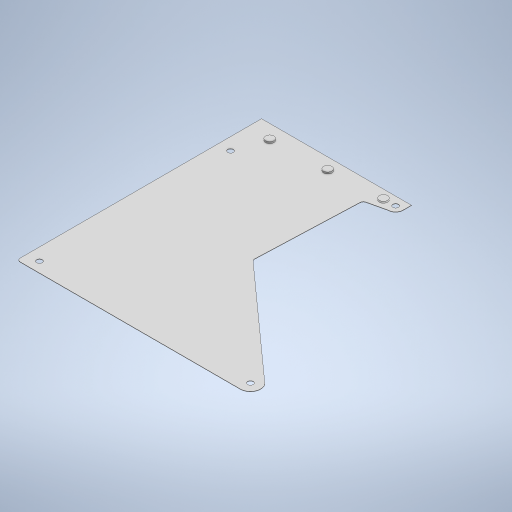
# Autodesk Inventor part: base_main_pcb_p1_itr2
Saved by Autodesk Inventor 2024 (Build 280153000, 153)
## iProperties
Created: 2026-03-21
Part Number: base_main_pcb_p1_itr2
Material: Generic
Document SubType Name: Modeling
Designer: schar
Density: 1 g/cm^3
Appearance: Default
Author: schar
Autodesk Inventor part; units mm, degrees
ref_plane "YZ Plane" through (0, 0, 0) normal (1, 0, 0) x (0, 1, 0)
ref_plane "XZ Plane" through (0, 0, 0) normal (0, 1, 0) x (-1, 0, 0)
ref_plane "XY Plane" through (0, 0, 0) normal (0, 0, 1) x (1, 0, 0)
ref_plane "Work Plane1" through (-203, 0.4, 290) normal (0, 1, 0) x (1, 0, 0)
sketch "Sketch1" plane through (-203, 0.4, 290) normal (0, 1, 0) x (1, 0, 0)
  arc A0 (133.6, 0) -> (138.4129, 10.1472) centre (133.6, 6.215) ccw projected
  circle A1 centre (133.6, 6.215) radius 1.675 projected
  circle A2 centre (133.6, 6.215) radius 1.675 projected
  circle A3 centre (133.6, 6.215) radius 1.675 projected
  circle A4 centre (133.6, 6.215) radius 1.675 projected
  arc A5 (133.6, 0) -> (138.4129, 10.1472) centre (133.6, 6.215) ccw projected
  arc A6 (133.6, 0) -> (138.4129, 10.1472) centre (133.6, 6.215) ccw projected
  arc A7 (133.6, 0) -> (138.4129, 10.1472) centre (133.6, 6.215) ccw projected
  circle A8 centre (84.5, 143.475) radius 1.675 projected
  arc A9 (84.5, 138.975) -> (89, 143.475) centre (84.5, 143.475) ccw projected
  arc A10 (73.455, 136.4093) -> (71.909, 134.5363) centre (73.9075, 134.4612) ccw projected
  arc A11 (73.455, 136.4093) -> (71.909, 134.5363) centre (73.9075, 134.4612) ccw projected
  circle A12 centre (5.5, 122.225) radius 1.675 projected
  circle A13 centre (5.5, 122.225) radius 1.675 projected
  circle A14 centre (5.5, 122.225) radius 1.675 projected
  circle A15 centre (5.5, 122.225) radius 1.675 projected
  line L0 (69.5853, 72.7034) -> (71.909, 134.5363) projected
  line L1 (69.5853, 72.7034) -> (71.909, 134.5363) projected
  line L2 (69.5853, 72.7034) -> (71.909, 134.5363) projected
  line L3 (69.5853, 72.7034) -> (71.909, 134.5363) projected
  circle A16 centre (5.5, 6.215) radius 1.675 projected
  line L4 (0, 0) -> (133.6, 0) projected
  line L5 (0, 0) -> (133.6, 0) projected
  line L6 (0, 0) -> (133.6, 0) projected
  line L7 (0, 0) -> (133.6, 0) projected
  line L8 (138.4129, 10.1472) -> (70.2502, 71.1379) projected
  line L9 (138.4129, 10.1472) -> (70.2502, 71.1379) projected
  line L10 (138.4129, 10.1472) -> (70.2502, 71.1379) projected
  line L11 (138.4129, 10.1472) -> (70.2502, 71.1379) projected
  arc A17 (73.455, 136.4093) -> (71.909, 134.5363) centre (73.9075, 134.4612) ccw projected
  arc A18 (73.455, 136.4093) -> (71.909, 134.5363) centre (73.9075, 134.4612) ccw projected
  circle A19 centre (5.5, 6.215) radius 1.675 projected
  arc A20 (-2, 2) -> (0, 0) centre (0, 2) ccw projected
  arc A21 (-2, 2) -> (0, 0) centre (0, 2) ccw projected
  arc A22 (-2, 2) -> (0, 0) centre (0, 2) ccw projected
  arc A23 (-2, 2) -> (0, 0) centre (0, 2) ccw projected
  circle A24 centre (5.5, 6.215) radius 1.675 projected
  circle A25 centre (5.5, 6.215) radius 1.675 projected
  arc A26 (69.5853, 72.7034) -> (70.2502, 71.1379) centre (71.5839, 72.6283) ccw projected
  arc A27 (69.5853, 72.7034) -> (70.2502, 71.1379) centre (71.5839, 72.6283) ccw projected
  arc A28 (69.5853, 72.7034) -> (70.2502, 71.1379) centre (71.5839, 72.6283) ccw projected
  arc A29 (69.5853, 72.7034) -> (70.2502, 71.1379) centre (71.5839, 72.6283) ccw projected
  arc A30 (84.5, 138.975) -> (89, 143.475) centre (84.5, 143.475) ccw projected
  circle A31 centre (84.5, 143.475) radius 1.675 projected
  circle A32 centre (84.5, 143.475) radius 1.675 projected
  circle A33 centre (84.5, 143.475) radius 1.675 projected
  arc A34 (84.5, 138.975) -> (89, 143.475) centre (84.5, 143.475) ccw projected
  arc A35 (84.5, 138.975) -> (89, 143.475) centre (84.5, 143.475) ccw projected
  line L12 (73.455, 136.4093) -> (84.5, 138.975) projected
  line L13 (73.455, 136.4093) -> (84.5, 138.975) projected
  line L14 (73.455, 136.4093) -> (84.5, 138.975) projected
  line L15 (73.455, 136.4093) -> (84.5, 138.975) projected
  line L16 (-2, 2) -> (-2, 148.562)
  line L17 (-2, 272.9952) -> (-2, 2) projected
  line L18 (-2, 148.562) -> (89, 148.562)
  line L19 (89, 143.475) -> (89, 199.525) projected
  line L20 (89, 148.562) -> (89, 143.475)
  point P0 (203, 290)
  point P1 (-2, 2)
  constraints: 6 end point, 3 point on line, 1 perpendicular
extrude "Extrusion1" add sketch "Sketch1" along normal blind 0.2
ref_plane "Work Plane2" through (-203, 0.6, 290) normal (0, 1, 0) x (1, 0, 0)
sketch "Sketch2" plane through (-203, 0.6, 290) normal (0, 1, 0) x (1, 0, 0)
  line L0 (-2, 272.9952) -> (-2, 2) projected
  arc A0 (84.5, 138.975) -> (89, 143.475) centre (84.5, 143.475) ccw projected
  line L1 (-2, 139.0629) -> (89, 143.475)
  circle A1 centre (11.7945, 139.7317) radius 2.5
  circle A2 centre (77.6916, 142.9267) radius 2.5
  circle A3 centre (45.3956, 141.3608) radius 2.5
  point P0 (203, 290)
  dimension "d3" = 5
  dimension "d6" = 5
  dimension "d7" = 5
  constraints: 4 point on line, 3 centre point, 2 end point
  measures "d3" diameter of A1
  measures "d6" diameter of A2
  measures "d7" diameter of A3
extrude "Extrusion2" add sketch "Sketch2" along normal blind 1
body "Solid2"
